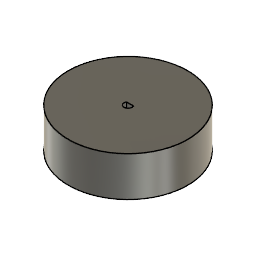
Wheel (Autodesk Fusion 360 design; units mm, degrees)
part number: 2026-04-02-18-33-10-450
Autodesk Fusion 360 part; units mm, degrees
sketch "Sketch1" plane through (0, 0, 0) normal (0, 0, 1) x (1, 0, 0)
  circle A0 centre (0, 0) radius 30
  circle A1 centre (0, 0) radius 2
  line L0 (-1.75, 0.9682) -> (1.75, 0.9682)
  dimension "d1" = 60
  dimension "d2" = 4
  dimension "d3" = 3.5
  constraint coincident A0.centre A1.centre
  constraint concentric A0 A1
  constraint coincident A1 L0.start
  constraint horizontal L0
  constraint coincident A1 L0.end
  measures "d1" diameter of A0
  measures "d2" diameter of A1
  measures "d3" distance of L0.start L0.end
extrude "Extrude1" add sketch "Sketch1" along normal blind 20 contours A0 | A1 L0 picked at (0.4695, 1.1188)
